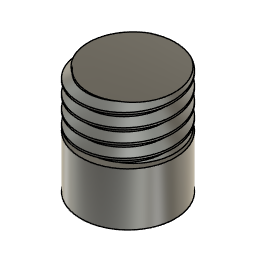
Bolt 20x18mm M2x2 (Autodesk Fusion 360 design; units mm, degrees)
Autodesk Fusion 360 part; units mm, degrees
sketch "Sketch1" plane through (0, 0, 0) normal (0, 0, 1) x (1, 0, 0)
  circle A0 centre (0, 0) radius 8.5
  dimension "d1" = 17
  constraint coincident A0.centre origin
  measures "d1" diameter of A0
extrude "Extrude1" add sketch "Sketch1" along normal blind 20
thread "Thread1" "ISO Metric profile 18.0 M18x2.5 6g" major diameter 17.7905 minor diameter 14.9379 pitch 2.5 angle 60 modelled right hand crest width 0.3601 on face at (8.4894, -0.4237, 13.3333) from (0, 0, 10) to (0, 0, 20) crest through (8.8953, 0, -0.625)
